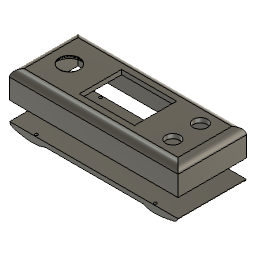
Gameboy1 (Autodesk Fusion 360 design; units mm, degrees)
part number: 2026-03-24-18-12-42-655
Autodesk Fusion 360 part; units mm, degrees
note: some values were not read from the file. Set by a fixed rule: which face or edge a step refers to.
sketch "Sketch1" plane through (0, 0, 0) normal (0, 0, 1) x (1, 0, 0)
  line L0 (32, 24.85) -> (-32, 24.85)
  line L1 (-32, 24.85) -> (-32, -24.85)
  line L2 (-32, -24.85) -> (32, -24.85)
  line L3 (32, -24.85) -> (32, 24.85)
  line L4 (32, 24.85) -> (-32, -24.85) construction
  line L5 (-32, 24.85) -> (32, -24.85) construction
  line L6 (32, 0) -> (64, 0) construction
  line L7 (-32, 0) -> (-64, 0) construction
  circle A0 centre (-64, 0) radius 11
  line L8 (64, 0) -> (92, 0) construction
  line L9 (-64, 0) -> (-92, 0) construction
  line L10 (0, 24.85) -> (0, 37.35) construction
  line L11 (0, -24.85) -> (0, -37.35) construction
  line L12 (92, 0) -> (92, -37.35) construction
  line L13 (-92, 0) -> (-92, 37.35) construction
  line L14 (-92, 37.35) -> (92, 37.35)
  line L15 (92, 37.35) -> (92, -37.35)
  line L16 (92, -37.35) -> (-92, -37.35)
  line L17 (-92, -37.35) -> (-92, 37.35)
  line L18 (-64, 0) -> (-64, 17) construction
  line L19 (-64, 17) -> (-50.5, 17) construction
  line L20 (-50.5, 17) -> (-77.5, 17) construction
  line L21 (-77.5, 17) -> (-77.5, -17) construction
  line L22 (-77.5, -17) -> (-50.5, -17) construction
  line L23 (-50.5, -17) -> (-50.5, 17) construction
  line L24 (-77.5, 17) -> (-74.3, 17) construction
  line L25 (-74.3, 17) -> (-74.3, 15.9) construction
  circle A1 centre (-74.025, 14.4) radius 1.525
  line L26 (-74.025, 14.4) -> (-75.55, 14.4) construction
  line L27 (-50.5, 17) -> (-54.2, 17) construction
  line L28 (-54.2, 17) -> (-54.2, 15.9) construction
  circle A2 centre (-54.1994, 14.375) radius 1.525
  line L29 (-54.1994, 14.375) -> (-54.1994, 12.85) construction
  line L30 (-54.1994, 12.85) -> (-54.1994, -10.3) construction
  circle A3 centre (-54.198, -11.825) radius 1.525
  line L31 (-74.3, 12.9) -> (-74.3, -10.25) construction
  circle A4 centre (-74.3, -11.775) radius 1.525
  line L32 (32, 24.85) -> (46.1, 24.85) construction
  line L33 (32, -24.85) -> (38.9, -24.85) construction
  line L34 (38.9, -24.85) -> (35.8, -24.85) construction
  line L35 (35.8, -24.85) -> (35.8, -23.55) construction
  line L36 (46.1, 24.85) -> (40.6, 24.85) construction
  line L37 (40.6, 24.85) -> (40.6, 23.85) construction
  circle A5 centre (40.5999, 22.325) radius 1.525
  line L38 (-32, 24.85) -> (-42.3, 24.85) construction
  line L39 (-42.3, 24.85) -> (-35.4, 24.85) construction
  line L40 (-35.4, 24.85) -> (-35.4, 23.85) construction
  circle A6 centre (-35.3999, 22.325) radius 1.525
  line L41 (-32, -24.85) -> (-42.3, -24.85) construction
  line L42 (-42.3, -24.85) -> (-35.4, -24.85) construction
  line L43 (-35.4, -24.85) -> (-35.4, -23.55) construction
  circle A7 centre (-35.4, -22.025) radius 1.525
  line L44 (64, 0) -> (64, 15) construction
  circle A8 centre (64, 15) radius 7.8
  circle A9 centre (64, -15) radius 7.8
  line L45 (40.5999, 22.325) -> (39.0749, 22.325) construction
  line L46 (-35.3999, 22.325) -> (-35.3999, 20.8) construction
  circle A10 centre (40.5999, -22.325) radius 1.525
  line L47 (40.5999, 22.325) -> (40.5999, 20.8) construction
  line L48 (-30, -23) -> (30, -23)
  line L49 (30, -23) -> (30, 23)
  line L50 (30, 23) -> (-30, 23)
  line L51 (-30, 23) -> (-30, -23)
  dimension "d6" = 64
  dimension "d7" = 49.7
  dimension "d8" = 32
  dimension "d10" = 32
  dimension "d11" = 22
  dimension "d12" = 28
  dimension "d13" = 28
  dimension "d14" = 12.5
  dimension "d15" = 12.5
  dimension "d33" = 17
  dimension "d34" = 13.5
  dimension "d35" = 27
  dimension "d36" = 34
  dimension "d37" = 3.2
  dimension "d38" = 1.1
  dimension "d39" = 3.05
  dimension "d40" = 3.7
  dimension "d41" = 1.1
  dimension "d42" = 3.05
  dimension "d43" = 23.15
  dimension "d44" = 3.05
  dimension "d45" = 23.15
  dimension "d46" = 3.05
  dimension "d47" = 14.1
  dimension "d48" = 6.9
  dimension "d49" = 3.1
  dimension "d50" = 1.3
  dimension "d52" = 5.5
  dimension "d53" = 1
  dimension "d54" = 3.05
  dimension "d55" = 10.3
  dimension "d56" = 6.9
  dimension "d57" = 1
  dimension "d58" = 3.05
  dimension "d59" = 10.3
  dimension "d60" = 6.9
  dimension "d61" = 1.3
  dimension "d62" = 3.05
  dimension "d90" = 15.6
  constraint horizontal L0
  constraint perpendicular L0 L1
  constraint parallel L0 L2
  constraint parallel L1 L3
  constraint coincident L4 origin
  constraint coincident L5 origin
  constraint midpoint L3 L6.start
  constraint perpendicular L3 L6
  constraint midpoint L1 L7.start
  constraint perpendicular L1 L7
  constraint coincident L7.end A0.centre
  constraint parallel L6 L8
  constraint parallel L7 L9
  constraint midpoint L0 L10.start
  constraint perpendicular L0 L10
  constraint midpoint L2 L11.start
  constraint perpendicular L2 L11
  constraint perpendicular L8 L12
  constraint horizontal L11.end L12.end
  constraint perpendicular L9 L13
  constraint horizontal L10.end L13.end
  constraint horizontal L14
  constraint vertical L15
  constraint horizontal L16
  constraint vertical L17
  constraint perpendicular L7 L18
  constraint perpendicular L18 L19
  constraint horizontal L20
  constraint vertical L21
  constraint horizontal L22
  constraint vertical L23
  constraint perpendicular L21 L24
  constraint perpendicular L20 L25
  constraint coincident L25.end A1
  constraint coincident A1.centre L26.start
  constraint coincident A1 L26.end
  constraint perpendicular L21 L26
  constraint perpendicular L23 L27
  constraint perpendicular L27 L28
  constraint coincident L28.end A2
  constraint coincident A2.centre L29.start
  constraint coincident A2 L29.end
  constraint perpendicular L20 L29
  constraint perpendicular L20 L30
  constraint coincident L30.end A3
  constraint coincident A1 L31.start
  constraint perpendicular L26 L31
  constraint coincident L31.end A4
  constraint perpendicular L3 L32
  constraint perpendicular L3 L33
  constraint parallel L33 L34
  constraint perpendicular L33 L35
  constraint parallel L32 L36
  constraint perpendicular L36 L37
  constraint coincident L37.end A5
  constraint perpendicular L1 L38
  constraint parallel L38 L39
  constraint perpendicular L38 L40
  constraint coincident L40.end A6
  constraint perpendicular L1 L41
  constraint perpendicular L23 L42
  constraint perpendicular L41 L43
  constraint coincident L43.end A7
  constraint perpendicular L8 L44
  constraint coincident L44.end A8.centre
  constraint symmetric L6 A8 A9
  constraint coincident A5.centre L45.start
  constraint coincident A5 L45.end
  constraint perpendicular L3 L45
  constraint coincident A6.centre L46.start
  constraint coincident A6 L46.end
  constraint parallel L1 L46
  constraint symmetric L6 A5 A10
  constraint coincident A5 L47.end
  constraint perpendicular L45 L47
  constraint horizontal L48
  constraint vertical L49
  constraint horizontal L50
  constraint vertical L51
  measures "d6" distance of L1.end L2.end
  measures "d7" distance of L0.end L1.end
  measures "d8" distance of L6.start L6.end
  measures "d10" distance of L7.start L7.end
  measures "d11" diameter of A0
  measures "d12" distance of L6.end L8.end
  measures "d13" distance of L7.end L9.end
  measures "d14" distance of L10.start L10.end
  measures "d15" distance of L11.start L11.end
  measures "d33" distance of L7.end L18.end
  measures "d34" distance of L18.end L19.end
  measures "d35" distance of L19.end L20.end
  measures "d36" distance of L19.end L22.end
  measures "d37" distance of L20.end L24.end
  measures "d38" distance of L24.end L25.end
  measures "d39" diameter of A1
  measures "d40" distance of L19.end L27.end
  measures "d41" distance of L27.end L28.end
  measures "d42" diameter of A2
  measures "d43" distance of L29.end L30.end
  measures "d44" diameter of A3
  measures "d45" distance of L31.start L31.end
  measures "d46" diameter of A4
  measures "d47" distance of L0.start L32.end
  measures "d48" distance of L2.end L33.end
  measures "d49" distance of L33.end L34.end
  measures "d50" distance of L34.end L35.end
  measures "d52" distance of L32.end L36.end
  measures "d53" distance of L36.end L37.end
  measures "d54" diameter of A5
  measures "d55" distance of L0.end L38.end
  measures "d56" distance of L38.end L39.end
  measures "d57" distance of L39.end L40.end
  measures "d58" diameter of A6
  measures "d59" distance of L1.end L41.end
  measures "d60" distance of L41.end L42.end
  measures "d61" distance of L42.end L43.end
  measures "d62" diameter of A7
  measures "d90" diameter of A8
extrude "Extrude1" add sketch "Sketch1" along normal blind 6 contours L14 L15 L16 L17 | A1 | A2 | A3 | A4 | A5 | A6 | A7 | A8 | A9 | A10 makes body 1
sketch "Sketch5" plane through (0, 37.35, 0) normal (0, 1, 0) x (-1, 0, 0)
  line L0 (-92, 0) -> (92, 0)
  line L1 (92, 0) -> (92, 6)
  line L2 (92, 6) -> (-92, 6)
  line L3 (-92, 6) -> (-92, 0)
  line L4 (-92, 0) -> (92, 0)
  line L5 (92, 0) -> (92, -50)
  line L6 (92, -50) -> (-92, -50)
  line L7 (-92, -50) -> (-92, 0)
  dimension "d19" = 50
  constraint horizontal L4
  constraint vertical L5
  constraint horizontal L6
  constraint vertical L7
  constraint coincident L0.start L3.end
  measures "d19" distance of L0.start L6.end
extrude "Extrude2" add sketch "Sketch5" against normal blind 5 contours L0 L4 L5 L6 L7 bodies 1
sketch "Sketch6" plane through (0, -37.35, 0) normal (0, -1, 0) x (1, 0, 0)
  line L0 (-92, 0) -> (92, 0)
  line L1 (92, 0) -> (92, 6)
  line L2 (92, 6) -> (-92, 6)
  line L3 (-92, 6) -> (-92, 0)
  line L4 (-92, 0) -> (92, 0)
  line L5 (92, 0) -> (92, -50)
  line L6 (92, -50) -> (-92, -50)
  line L7 (-92, -50) -> (-92, 0)
  dimension "d22" = 50
  constraint horizontal L4
  constraint vertical L5
  constraint horizontal L6
  constraint vertical L7
  constraint coincident L0.start L3.end
  measures "d22" distance of L0.start L6.end
extrude "Extrude3" add sketch "Sketch6" against normal blind 5 contours L0 L4 L5 L6 L7 bodies 1
sketch "Sketch7" plane through (92, 0, 0) normal (1, 0, 0) x (0, 1, 0)
  line L0 (37.35, -50) -> (37.35, 6)
  line L1 (37.35, 6) -> (-37.35, 6)
  line L2 (-37.35, 6) -> (-37.35, -50)
  line L3 (-37.35, -50) -> (-32.35, -50)
  line L4 (-32.35, -50) -> (-32.35, 0)
  line L5 (-32.35, 0) -> (32.35, 0)
  line L6 (32.35, 0) -> (32.35, -50)
  line L7 (32.35, -50) -> (37.35, -50)
sketch "Sketch8" plane through (92, 0, 0) normal (1, 0, 0) x (0, 1, 0)
  line L0 (-32.35, -50) -> (32.35, -50)
  line L1 (32.35, -50) -> (32.35, 0)
  line L2 (32.35, 0) -> (-32.35, 0)
  line L3 (-32.35, 0) -> (-32.35, -50)
  constraint horizontal L0
  constraint vertical L1
  constraint horizontal L2
  constraint vertical L3
extrude "Extrude4" add sketch "Sketch8" against normal blind 5 bodies 1
sketch "Sketch9" plane through (-92, 0, 0) normal (-1, 0, 0) x (0, -1, 0)
  line L0 (37.35, -50) -> (37.35, 6)
  line L1 (37.35, 6) -> (-37.35, 6)
  line L2 (-37.35, 6) -> (-37.35, -50)
  line L3 (-37.35, -50) -> (-32.35, -50)
  line L4 (-32.35, -50) -> (-32.35, 0)
  line L5 (-32.35, 0) -> (32.35, 0)
  line L6 (32.35, 0) -> (32.35, -50)
  line L7 (32.35, -50) -> (37.35, -50)
  line L8 (-32.35, 0) -> (32.35, 0)
  line L9 (32.35, 0) -> (32.35, -50)
  line L10 (32.35, -50) -> (-32.35, -50)
  line L11 (-32.35, -50) -> (-32.35, 0)
  constraint horizontal L8
  constraint vertical L9
  constraint horizontal L10
  constraint vertical L11
  constraint coincident L6.end L7.start
  constraint coincident L4.end L5.start
extrude "Extrude5" add sketch "Sketch9" against normal blind 5 contours L4 L5 L6 L8 L9 L10 L11 bodies 1
sketch "Sketch10" plane through (-92, 0, 0) normal (-1, 0, 0) x (0, -1, 0)
  line L0 (37.35, -50) -> (37.35, 6)
  line L1 (37.35, 6) -> (-37.35, 6)
  line L2 (-37.35, 6) -> (-37.35, -50)
  line L3 (-37.35, -50) -> (37.35, -50)
  line L4 (-25, -50) -> (-11, -50)
  line L5 (-11, -50) -> (-11, -43)
  line L6 (-11, -43) -> (-25, -43)
  line L7 (-25, -43) -> (-25, -50)
  constraint horizontal L4
  constraint vertical L5
  constraint horizontal L6
  constraint vertical L7
  constraint coincident L3 L4.start
extrude "Extrude6" cut sketch "Sketch10" against normal blind 5 contours L3 L4 L5 L6 L7 bodies 1
sketch "Sketch11" plane through (0, 0, 6) normal (0, 0, 1) x (-1, 0, 0)
  circle A0 centre (64, 0) radius 11
  line L0 (-32, -24.85) -> (-32, 24.85)
  line L1 (-32, 24.85) -> (32, 24.85)
  line L2 (32, 24.85) -> (32, -24.85)
  line L3 (32, -24.85) -> (-32, -24.85)
  line L4 (92, 37.35) -> (-92, 37.35)
  line L5 (-92, 37.35) -> (-92, -37.35)
  line L6 (-92, -37.35) -> (92, -37.35)
  line L7 (92, -37.35) -> (92, 37.35)
extrude "Extrude7" cut sketch "Sketch11" against normal blind 5 bodies 1
extrude "Extrude8" add sketch "Sketch1" along normal blind 5 contours L14 L15 L16 L17 | A8 | A9 | A10 bodies 1
sketch "Sketch12" plane through (0, 0, -50) normal (0, 0, -1) x (1, 0, 0)
  line L0 (92, 37.35) -> (-92, 37.35)
  line L1 (-92, 37.35) -> (-92, -11)
  line L2 (-92, -11) -> (-87, -11)
  line L3 (-87, -11) -> (-87, 32.35)
  line L4 (-87, 32.35) -> (87, 32.35)
  line L5 (87, 32.35) -> (87, -32.35)
  line L6 (87, -32.35) -> (-87, -32.35)
  line L7 (-87, -32.35) -> (-87, -25)
  line L8 (-87, -25) -> (-92, -25)
  line L9 (-92, -25) -> (-92, -37.35)
  line L10 (-92, -37.35) -> (92, -37.35)
  line L11 (92, -37.35) -> (92, 32.35)
  line L12 (-87, 32.35) -> (-89, 32.35) construction
  line L13 (-89, 32.35) -> (-89, 34.85) construction
  line L14 (-87, 32.35) -> (-87, 35) construction
  line L15 (-86.7, 34.85) -> (-87.85, 36.8419)
  line L16 (-87.85, 36.8419) -> (-90.15, 36.8419)
  line L17 (-90.15, 36.8419) -> (-91.3, 34.85)
  line L18 (-91.3, 34.85) -> (-90.15, 32.8581)
  line L19 (-90.15, 32.8581) -> (-87.85, 32.8581)
  line L20 (-87.85, 32.8581) -> (-86.7, 34.85)
  line L21 (92, 32.35) -> (92, 37.35)
  point P0 (-89, 34.85)
  dimension "d69" = 2
  dimension "d70" = 2.5
  dimension "d71" = 2.3
  constraint coincident L3.end L4.start
  constraint perpendicular L1 L12
  constraint perpendicular L0 L13
  constraint perpendicular L4 L14
  constraint coincident P0 L13.end
  measures "d69" distance of L3.end L12.end
  measures "d70" distance of L12.end P0
  measures "d71" distance of L15.start P0
extrude "Extrude9" cut sketch "Sketch12" against normal blind 14 contours L15 L16 L17 L18 L19 L20 bodies 1
sketch "Sketch13" plane through (0, 0, -50) normal (0, 0, -1) x (1, 0, 0)
  line L0 (-87.85, 36.8419) -> (-86.7, 34.85)
  line L1 (-86.7, 34.85) -> (-87.85, 32.8581)
  line L2 (-87.85, 32.8581) -> (-90.15, 32.8581)
  line L3 (-90.15, 32.8581) -> (-91.3, 34.85)
  line L4 (-91.3, 34.85) -> (-90.15, 36.8419)
  line L5 (-90.15, 36.8419) -> (-87.85, 36.8419)
  line L6 (92, 37.35) -> (-92, 37.35)
  line L7 (-92, 37.35) -> (-92, -11)
  line L8 (-92, -11) -> (-87, -11)
  line L9 (-87, -11) -> (-87, 32.35)
  line L10 (-87, 32.35) -> (87, 32.35)
  line L11 (87, 32.35) -> (87, -32.35)
  line L12 (87, -32.35) -> (-87, -32.35)
  line L13 (-87, -32.35) -> (-87, -25)
  line L14 (-87, -25) -> (-92, -25)
  line L15 (-92, -25) -> (-92, -37.35)
  line L16 (-92, -37.35) -> (92, -37.35)
  line L17 (92, -37.35) -> (92, 32.35)
  line L18 (87, 32.35) -> (89, 32.35) construction
  line L19 (89, 32.35) -> (89, 34.85) construction
  line L20 (87, 32.35) -> (87, 35) construction
  line L21 (86.7, 34.85) -> (87.85, 32.8581)
  line L22 (87.85, 32.8581) -> (90.15, 32.8581)
  line L23 (90.15, 32.8581) -> (91.3, 34.85)
  line L24 (91.3, 34.85) -> (90.15, 36.8419)
  line L25 (90.15, 36.8419) -> (87.85, 36.8419)
  line L26 (87.85, 36.8419) -> (86.7, 34.85)
  line L27 (92, 0) -> (86, 0) construction
  line L28 (90.15, -36.8419) -> (87.85, -36.8419)
  line L29 (87.85, -36.8419) -> (86.7, -34.85)
  line L30 (86.7, -34.85) -> (87.85, -32.8581)
  line L31 (91.3, -34.85) -> (90.15, -36.8419)
  line L32 (90.15, -32.8581) -> (91.3, -34.85)
  line L33 (87.85, -32.8581) -> (90.15, -32.8581)
  line L34 (0, -33) -> (0, -36) construction
  line L35 (-87.85, -32.8581) -> (-90.15, -32.8581)
  line L36 (-86.7, -34.85) -> (-87.85, -32.8581)
  line L37 (-87.85, -36.8419) -> (-86.7, -34.85)
  line L38 (-90.15, -32.8581) -> (-91.3, -34.85)
  line L39 (-90.15, -36.8419) -> (-87.85, -36.8419)
  line L40 (-91.3, -34.85) -> (-90.15, -36.8419)
  arc A0 (-92, -36.35) -> (-91, -37.35) centre (-91, -36.35) ccw
  line L41 (-92, -36.35) -> (-91, -36.35) construction
  line L42 (-91, -36.35) -> (-91, -37.35) construction
  line L43 (-91, -37.35) -> (-92, -37.35) construction
  line L44 (-92, -37.35) -> (-92, -36.35) construction
  line L45 (91, 37.35) -> (92, 37.35) construction
  line L46 (92, 37.35) -> (92, 36.35) construction
  line L47 (92, 36.35) -> (91, 36.35) construction
  line L48 (91, 36.35) -> (91, 37.35) construction
  line L49 (92, 37.35) -> (-92, 37.35)
  line L50 (-92, 37.35) -> (-92, -37.35)
  line L51 (-92, -37.35) -> (92, -37.35)
  line L52 (92, -37.35) -> (92, 37.35)
  circle A1 centre (89, 34.85) radius 1.5
  circle A2 centre (89, -34.85) radius 1.5
  circle A3 centre (-89, 34.85) radius 1.5
  circle A4 centre (-89, -34.85) radius 1.5
  line L53 (92, 32.35) -> (92, 37.35)
  point P0 (89, 34.85)
  point P1 (-91, -36.35)
  dimension "d74" = 2
  dimension "d75" = 2.5
  dimension "d76" = 2.3
  dimension "d81" = 3
  constraint coincident L10.end L11.start
  constraint perpendicular L17 L18
  constraint perpendicular L18 L19
  constraint perpendicular L10 L20
  constraint coincident P0 L19.end
  constraint midpoint L17 L27.start
  constraint perpendicular L11 L27
  constraint symmetric L21.start L27 L29.end
  constraint symmetric L21.end L27 L30.end
  constraint symmetric L22.end L27 L32.start
  constraint symmetric L23.end L27 L31.start
  constraint symmetric L24.end L27 L28.start
  constraint symmetric L25.end L27 L28.end
  constraint vertical L34
  constraint symmetric L28.start L34 L39.start
  constraint symmetric L28.end L34 L37.start
  constraint symmetric L29.end L34 L36.start
  constraint symmetric L30.end L34 L35.start
  constraint symmetric L31.start L34 L38.end
  constraint symmetric L32.start L34 L35.end
  constraint horizontal L41
  constraint vertical L42
  constraint horizontal L43
  constraint vertical L44
  constraint coincident A0.end L42.end
  constraint coincident A0.start L41.start
  constraint horizontal L45
  constraint vertical L46
  constraint horizontal L47
  constraint vertical L48
  constraint coincident L17.end L46.end
  constraint coincident L6.start L45.start
  constraint horizontal L49
  constraint vertical L50
  constraint horizontal L51
  constraint vertical L52
  constraint symmetric L27 A1 A2
  constraint symmetric L34 A1 A3
  constraint symmetric L27 A3 A4
  measures "d74" distance of L10.end L18.end
  measures "d75" distance of L18.end P0
  measures "d76" distance of L21.start P0
  measures "d81" diameter of A1
extrude "Extrude10" cut sketch "Sketch13" against normal blind 14 contours L35 L36 L37 L38 L39 L40 | A4 bodies 1
extrude "Extrude11" cut sketch "Sketch13" against normal blind 14 contours L21 L22 L23 L24 L25 L26 | L28 L29 L30 L31 L32 L33 | A1 | A2 bodies 1
sketch "Sketch14" plane through (0, 0, -50) normal (0, 0, -1) x (1, 0, 0)
extrude "Extrude13" cut 1 faces at (-34.3431, -22.132, 1) along direction (0, 0, -1) blind 1 on bodies 1 bodies 1
extrude "Extrude14" cut 7 faces at (-55.2549, -11.6324, 1) (-73.6842, -12.1948, 1) (-73.4092, 13.9802, 1) (-55.2562, 14.5676, 1) (-34.3431, 22.218, 1) (41.594, 22.1752, 1) (-73.6842, -12.1948, 1) along direction (0, 0, -1) blind 1 on bodies 1 bodies 1
extrude "Extrude15" cut sketch "Sketch1" along normal blind 5 contours A8 bodies 1
extrude "Extrude16" cut sketch "Sketch1" along normal blind 5 contours A9 bodies 1
form "Form1" [no effect]
sketch "Sketch15" plane through (0, 0, 0) normal (0, 0, -1) x (1, 0, 0)
  circle A0 centre (64, 15) radius 7.8
  circle A1 centre (64, -15) radius 7.8
  circle A2 centre (40.5999, -22.325) radius 1.525
  circle A3 centre (-54.1994, -14.375) radius 1.525
  circle A4 centre (-74.3, 11.775) radius 1.525
  circle A5 centre (-54.198, 11.825) radius 1.525
  circle A6 centre (-74.025, -14.4) radius 1.525
  circle A7 centre (-35.3999, -22.325) radius 1.525
  circle A8 centre (-64, 0) radius 11
  line L0 (32, 24.85) -> (32, -24.85)
  line L1 (32, -24.85) -> (-32, -24.85)
  line L2 (-32, -24.85) -> (-32, 24.85)
  line L3 (-32, 24.85) -> (32, 24.85)
  line L4 (-87, 32.35) -> (-87, -32.35)
  line L5 (-87, -32.35) -> (87, -32.35)
  line L6 (87, -32.35) -> (87, 32.35)
  line L7 (87, 32.35) -> (-87, 32.35)
  circle A9 centre (-35.4, 22.025) radius 1.525
pipe "Pipe1" cut diameter 6 along 1 edges at (-75, 0, 0) on bodies 1 bodies 1
fillet "Fillet4" radius 2 1 edges at (-74.2556, 3.9778, 3) on bodies 1
extrude "Extrude17" cut 3 faces at (-89.7167, 27.6194, -50) (-88.6667, -3.45, -50) (88.6667, 10.7833, -50) along direction (0, 0, 1) blind 40 on bodies 1 bodies 1
extrude "Extrude18" cut 4 faces at (89.3833, -34.186, -36) (89.3833, 34.186, -36) (-88.6167, 35.514, -36) (-88.6167, -34.186, -36) along direction (0, 0, 1) blind 26 on bodies 1 bodies 1
extrude "Extrude19" cut 1 faces at (-90.3333, 15.6667, -43) along direction (0, 0, 1) blind 33 on bodies 1 bodies 1
sketch "Sketch16" plane through (0, 37.35, 0) normal (0, 1, 0) x (-1, 0, 0)
  line L0 (-92, -10) -> (92, -10)
  line L1 (92, -10) -> (92, 5)
  line L2 (92, 5) -> (-92, 5)
  line L3 (-92, 5) -> (-92, -10)
extrude "Extrude20" add 4 faces at (-29, 35.6833, -10) (-29, -35.6833, -10) (-90.3333, 15.6667, -10) (88.6667, 10.7833, -10) along direction (0, 0, -1) blind 15 on bodies 1 bodies 1
fillet "Fillet5" radius 8 4 edges at (92, 0, 5) (0, -37.35, 5) (-92, 0, 5) (0, 37.35, 5) on bodies 1
sketch "Sketch17" plane through (0, 0, -25) normal (0, 0, 1) x (1, 0, 0)
  line L0 (92, 37.35) -> (-92, 37.35)
  line L1 (-92, 37.35) -> (-92, -37.35)
  line L2 (-92, -37.35) -> (92, -37.35)
  line L3 (92, -37.35) -> (92, 37.35)
  line L4 (87, 32.35) -> (77, 32.35) construction
  line L5 (77, 32.35) -> (77, 37.35) construction
  circle A0 centre (77, 34.85) radius 1.65
  line L6 (-2.3799, 0) -> (4, 0) construction
  line L7 (0, 3) -> (0, -5) construction
  circle A1 centre (-77, 34.85) radius 1.65
  circle A2 centre (77, -34.85) radius 1.65
  circle A3 centre (-77, -34.85) radius 1.65
  line L8 (-92, -37.35) -> (-92, 37.35)
  line L9 (-92, 37.35) -> (92, 37.35)
  line L10 (92, 37.35) -> (92, -37.35)
  line L11 (92, -37.35) -> (-92, -37.35)
  line L12 (-87, 32.35) -> (-87, -32.35)
  line L13 (-87, -32.35) -> (87, -32.35)
  line L14 (87, -32.35) -> (87, 32.35)
  line L15 (87, 32.35) -> (-87, 32.35)
  point P0 (92, 37.35)
  point P1 (-92, -37.35)
  point P2 (87, 32.35)
  dimension "d111" = 3.3
  constraint horizontal L0
  constraint vertical L1
  constraint horizontal L2
  constraint vertical L3
  constraint coincident P2 L4.start
  constraint parallel L0 L4
  constraint coincident L0 L5.end
  constraint perpendicular L0 L5
  constraint midpoint L5 A0.centre
  constraint perpendicular L3 L6
  constraint vertical L7
  constraint symmetric A0 L7 A1
  constraint symmetric A0 L6 A2
  constraint symmetric L6 A1 A3
  measures "d111" diameter of A0
extrude "Extrude43" cut sketch "Sketch1" along normal blind 5 contours A10 bodies 1
sketch "Sketch23" plane through (0, 0, 0) normal (0, 0, 1) x (1, 0, 0)
extrude "Extrude44" add sketch "Sketch1" along normal blind 5 contours L0 L1 L2 L3 bodies 1
sketch "Sketch24" plane through (0, 37.35, 0) normal (0, 1, 0) x (-1, 0, 0)
  line L0 (92, -3) -> (-92, -3)
  line L1 (-92, -3) -> (-92, -25)
  line L2 (-92, -25) -> (92, -25)
  line L3 (92, -25) -> (92, -3)
  line L4 (-92, -3) -> (-86, -3) construction
  line L5 (-86, -3) -> (-86, -5) construction
  line L6 (-86, -5) -> (-72.2, -5)
  line L7 (-72.2, -5) -> (-72.2, -17.5)
  line L8 (-72.2, -17.5) -> (-86, -17.5)
  line L9 (-86, -17.5) -> (-86, -5)
  line L10 (-86, -10) -> (-72.2, -10)
  line L11 (-72.2, -10) -> (-72.2, -11.9724)
  line L12 (-72.2, -11.9724) -> (-86, -11.9724)
  line L13 (-86, -11.9724) -> (-86, -10)
  dimension "d168" = 13.8
  dimension "d169" = 12.5
  constraint coincident L0.end L1.start
  constraint coincident L0 L4.end
  constraint perpendicular L4 L5
  constraint horizontal L6
  constraint vertical L7
  constraint horizontal L8
  constraint vertical L9
  constraint horizontal L10
  constraint vertical L11
  constraint horizontal L12
  constraint vertical L13
  constraint coincident L7 L11.end
  constraint coincident L9 L10.start
  measures "d168" distance of L5.end L6.end
  measures "d169" distance of L5.end L8.end
extrude "Extrude45" cut sketch "Sketch24" against normal blind 5 contours L6 L7 L9 L10 bodies 1
extrude "Extrude46" cut sketch "Sketch24" against normal blind 5 contours L7 L8 L9 L12 bodies 1
extrude "Extrude47" add sketch "Sketch24" against normal blind 7 contours L7 L9 L10 L11 L12 L13 bodies 1
extrude "Extrude48" cut sketch "Sketch24" against normal blind 4.4 contours L7 L9 L10 L11 L12 L13 bodies 1
extrude "Extrude49" add 1 faces at (86, 31.6833, -11.3149) along direction (1, 0, 0) blind 1 on bodies 1 bodies 1
extrude "Extrude50" add 1 faces at (72.2, 31.6833, -10.6575) along direction (-1, 0, 0) blind 3 on bodies 1 bodies 1
sketch "Sketch25" plane through (0, 0, -25) normal (0, 0, -1) x (1, 0, 0)
  line L0 (-92, 37.35) -> (-92, -37.35)
  line L1 (-92, -37.35) -> (92, -37.35)
  line L2 (92, -37.35) -> (92, 37.35)
  line L3 (92, 37.35) -> (-92, 37.35)
  line L4 (-87, -32.35) -> (-87, 32.35)
  line L5 (-87, 32.35) -> (87, 32.35)
  line L6 (87, 32.35) -> (87, -32.35)
  line L7 (87, -32.35) -> (-87, -32.35)
  line L8 (-92, 37.35) -> (92, 37.35)
  line L9 (92, 37.35) -> (92, -37.35)
  line L10 (92, -37.35) -> (-92, -37.35)
  line L11 (-92, -37.35) -> (-92, 37.35)
  circle A0 centre (-65, 35) radius 1.525
  line L12 (0, 0) -> (0, 3.6241) construction
  line L13 (0, 0) -> (-25, 0) construction
  circle A1 centre (65, 35) radius 1.525
  circle A2 centre (65, -35) radius 1.525
  circle A3 centre (-65, -35) radius 1.525
  point P0 (-65, -35)
  dimension "d182" = 3.05
  dimension "d183" = 3.05
  constraint horizontal L8
  constraint vertical L9
  constraint horizontal L10
  constraint vertical L11
  constraint coincident L1.end L2.start
  constraint coincident L0.start L3.end
  constraint coincident L12.start L13.start
  constraint vertical L12
  constraint perpendicular L12 L13
  constraint symmetric A0 L12 A1
  constraint symmetric A0.centre L13 P0
  constraint symmetric L13 A1 A2
  constraint coincident P0 A3.centre
  measures "d182" diameter of A0
  measures "d183" diameter of A3
extrude "Extrude51" add sketch "Sketch25" along normal blind 5 separate body contours L0 L1 L2 L3 L8 L9 L10 L11 | L4 L5 L6 L7 makes body 2
move_body "Move5" bodies 2 to x (1, 0, 0) y (0, 1, 0) z (0, 0, 1) at (0, -30, 0)
move_body "Move6" bodies 2 to x (1, 0, 0) y (0, 1, 0) z (0, 0, 1) at (0, 30, -20)
fillet "Fillet7" radius 7 2 edges at (-92, 0, -50) (92, 0, -50) on bodies 2
sketch "Sketch26" plane through (0, 37.35, 0) normal (0, 1, 0) x (-1, 0, 0)
  arc A0 (-92, -45) -> (-85.2918, -50) centre (-85.2918, -43) ccw
  line L0 (-85.2918, -50) -> (85.2918, -50)
  arc A1 (85.2918, -50) -> (92, -45) centre (85.2918, -43) ccw
  line L1 (92, -45) -> (-92, -45)
  spline S0 degree 5 poles (-85.2918, -50) (-84.4956, -50.1956) (-82.9162, -50.5707) (-80.5867, -51.0846) (-77.5608, -51.6711) (-73.922, -52.2275) (-70.4414, -52.5889) (-67.136, -52.7345) (-64.0203, -52.6464) (-61.0976, -52.3207) (-58.3578, -51.7695) (-56.3026, -51.1602) (-54.8336, -50.6142) (-53.8858, -50.2112) (-53.4198, -50) knots 0 0 0 0 0 0 0.1 0.2 0.3 0.4 0.5 0.6 0.7 0.8 0.9 1 1 1 1 1 1
  line L2 (0, 0) -> (0, -8.4657) construction
  spline S1 degree 5 poles (85.2918, -50) (84.4956, -50.1956) (82.9162, -50.5707) (80.5867, -51.0846) (77.5608, -51.6711) (73.922, -52.2275) (70.4414, -52.5889) (67.136, -52.7345) (64.0203, -52.6464) (61.0976, -52.3207) (58.3578, -51.7695) (56.3026, -51.1602) (54.8336, -50.6142) (53.8858, -50.2112) (53.4198, -50) knots 0 0 0 0 0 0 0.1 0.2 0.3 0.4 0.5 0.6 0.7 0.8 0.9 1 1 1 1 1 1
  line L3 (-88.891, -49.1157) -> (-81.6925, -50.8843)
  line L4 (-56.144, -51.2349) -> (-50.6957, -48.7651)
  line L5 (88.891, -49.1157) -> (81.6925, -50.8843)
  line L6 (56.144, -51.2349) -> (50.6957, -48.7651)
  point P0 (-65.3611, -52.6534)
  point P1 (65.3611, -52.6534)
  constraint coincident A0.end L0.start
  constraint coincident L0 S0.end
  constraint coincident L2.start origin
  constraint perpendicular L1 L2
  constraint midpoint A0.end L3
  constraint midpoint S0.end L4
  constraint symmetric A0.end L2 L0.end
  constraint symmetric P0 L2 P1
  constraint symmetric S0.end L2 S1.end
  constraint symmetric L2 L3.start L5.start
  constraint symmetric L2 L3.end L5.end
  constraint symmetric L2 L4.start L6.start
  constraint symmetric L2 L4.end L6.end
extrude "Extrude52" add sketch "Sketch26" against normal blind 74.7 contours L0 S0 bodies 2
extrude "Extrude53" add sketch "Sketch26" against normal blind 74.7 contours L0 S1 bodies 2
extrude "Extrude54" cut sketch "Sketch25" along normal blind 50 contours A0 bodies 2
extrude "Extrude55" cut sketch "Sketch25" along normal blind 50 contours A1 | A2 | A3 bodies 2
extrude "Extrude56" cut sketch "Sketch25" against normal blind 6 contours A0 | A1 | A2 | A3 bodies 1
extrude "Extrude57" add sketch "Sketch1" along normal blind 5 contours A1 | A2 | A3 | A4 | A5 | A6 | A7 | A10 bodies 1
extrude "Extrude58" cut sketch "Sketch1" along normal blind 4 contours A1 | A2 | A3 | A4 | A5 | A6 | A7 | A10 bodies 1
extrude "Extrude59" add sketch "Sketch1" against normal blind 45 contours A0 bodies 2
extrude "Extrude60" cut sketch "Sketch1" against normal blind 40 contours A0 bodies 2
extrude "Extrude61" add 1 faces at (-65.7538, 6.6152, -40) along direction (0, 0, 1) blind 7 on bodies 2 bodies 2
extrude "Extrude21" [suppressed]
sketch "Sketch18" plane through (0, 0, 0) normal (0, 1, 0) x (1, 0, 0)
fillet "Fillet6" [suppressed]
sketch "Sketch19" plane through (0, -37.35, 0) normal (0, -1, 0) x (1, 0, 0)
  arc A0 (-92, -20) -> (-84.9289, -25) centre (-84.9289, -17.5) ccw
  line L0 (-84.9289, -25) -> (84.9289, -25)
  arc A1 (84.9289, -25) -> (92, -20) centre (84.9289, -17.5) ccw
  line L1 (92, -20) -> (-92, -20)
  line L2 (84.9289, -25) -> (49.9289, -25) construction
  spline S0 degree 2 poles (84.9289, -25) (62, -30) (49.9289, -25) knots 0 0 0 3.622646 3.622646 3.622646 weights 1 9 1
  line L3 (0, 0) -> (0, -32) construction
  spline S1 degree 2 poles (-84.9289, -25) (-62, -30) (-49.9289, -25) knots 0 0 0 3.622646 3.622646 3.622646 weights 1 9 1
  dimension "d116" = 35
  constraint coincident L0.end A1.start
  constraint parallel L0 L2
  constraint coincident L3.start origin
  constraint perpendicular L0 L3
  constraint symmetric L0.end L3 A0.end
  constraint symmetric L2.end L3 S1.end
  constraint symmetric S0 L3 S1
  measures "d116" distance of L0.end L2.end
extrude "Extrude22" [suppressed]
extrude "Extrude23" [suppressed]
extrude "Extrude24" [suppressed]
extrude "Extrude25" [suppressed]
extrude "Extrude26" [suppressed]
extrude "Extrude27" [suppressed]
move_body "Move2" [suppressed]
extrude "Extrude28" [suppressed]
sketch "Sketch20" plane through (0, 0, 0) normal (0, 1, 0) x (1, 0, 0)
sketch "Sketch21" plane through (0, 0, 0) normal (0, 0, 1) x (1, 0, 0)
sketch "Sketch22" plane through (0, 37.35, 0) normal (0, 1, 0) x (-1, 0, 0)
  line L0 (92, -3) -> (-92, -3)
  line L1 (-92, -3) -> (-92, -25)
  line L2 (-92, -25) -> (92, -25)
  line L3 (92, -25) -> (92, -3)
  line L4 (-92, -3) -> (-86, -3) construction
  line L5 (-86, -3) -> (-86, -4) construction
  line L6 (-86, -4) -> (-73, -4)
  line L7 (-73, -4) -> (-73, -16.2)
  line L8 (-73, -16.2) -> (-86, -16.2)
  line L9 (-86, -16.2) -> (-86, -4)
  line L10 (-86, -9) -> (-73, -9)
  line L11 (-73, -9) -> (-73, -11)
  line L12 (-73, -11) -> (-86, -11)
  line L13 (-86, -11) -> (-86, -9)
  dimension "d133" = 6
  dimension "d134" = 13
  dimension "d135" = 12.2
  constraint coincident L0.end L1.start
  constraint perpendicular L1 L4
  constraint perpendicular L0 L5
  constraint horizontal L6
  constraint vertical L7
  constraint horizontal L8
  constraint vertical L9
  constraint horizontal L10
  constraint vertical L11
  constraint horizontal L12
  constraint vertical L13
  constraint coincident L7 L11.end
  constraint coincident L9 L10.start
  measures "d133" distance of L0.end L4.end
  measures "d134" distance of L5.end L6.end
  measures "d135" distance of L5.end L8.end
extrude "Extrude29" [suppressed]
extrude "Extrude30" [suppressed]
extrude "Extrude31" [suppressed]
extrude "Extrude32" [suppressed]
extrude "Extrude33" [suppressed]
extrude "Extrude34" [suppressed]
extrude "Extrude35" [suppressed]
extrude "Extrude36" [suppressed]
extrude "Extrude37" [suppressed]
extrude "Extrude38" [suppressed]
extrude "Extrude39" [suppressed]
extrude "Extrude40" [suppressed]
extrude "Extrude41" [suppressed]
extrude "Extrude42" [suppressed]
move_body "Move3" [suppressed]
move_body "Move4" [suppressed]
equation "button_hole_diam = 15.6 mm"
equation "joy_hole_diam = 22 mm"
equation "lcd_height = 49.7 mm"
equation "lcd_width = 64 mm"
equation "thickness = 6 mm"
equation "d6 = lcd_width"
equation "d7 = lcd_height"
equation "d11 = joy_hole_diam"
equation "d16 = thickness"
equation "d34 = ( 27 / 2 ) * 1 mm"
equation "d37 = 1.7 mm + 1.5 mm"
equation "d40 = 2.2 mm + 1.5 mm"
equation "d117 = 0.9"
equation "d118 = d117"
